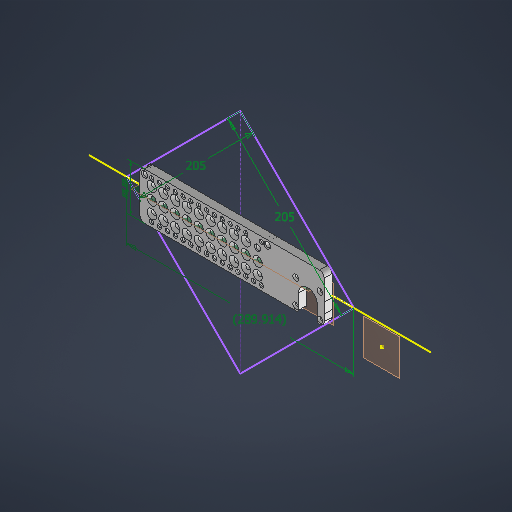
# Autodesk Inventor part: body2
Saved by Autodesk Inventor 2026.3 (Build 303398000, 398)
## iProperties
Created: 2026-04-19
Part Number: body2
Material: Generic
Document SubType Name: Modeling
Designer: micha
Density: 1 g/cm^3
Appearance: Default
Author: micha
Autodesk Inventor part; units mm, degrees
ref_plane "YZ Plane" through (0, 0, 0) normal (1, 0, 0) x (0, 1, 0)
ref_plane "XZ Plane" through (0, 0, 0) normal (0, 1, 0) x (-1, 0, 0)
ref_plane "XY Plane" through (0, 0, 0) normal (0, 0, 1) x (1, 0, 0)
ref_plane "Work Plane1" through (0, 0, 0) normal (0, 0, 1) x (1, 0, 0)
ref_plane "Work Plane2" through (-84.3749, 16.638, 0) normal (0, 0, 1) x (1, 0, 0)
sketch "Sketch2" plane through (-84.3749, 16.638, 0) normal (0, 0, 1) x (1, 0, 0)
  circle A0 centre (0, 0) radius 12
  arc A1 (21, 16.7929) -> (20.8536, 17.1464) centre (20.5, 16.7929) ccw projected
  line L0 (17.1464, 20.8536) -> (20.8536, 17.1464) projected
  arc A2 (17.1464, 20.8536) -> (16.7929, 21) centre (16.7929, 20.5) ccw projected
  line L1 (-16.7929, 21) -> (16.7929, 21) projected
  arc A3 (-16.7929, 21) -> (-17.1464, 20.8536) centre (-16.7929, 20.5) ccw projected
  line L2 (-20.8536, 17.1464) -> (-17.1464, 20.8536) projected
  arc A4 (-20.8536, 17.1464) -> (-21, 16.7929) centre (-20.5, 16.7929) ccw projected
  line L3 (-21, -16.7929) -> (-21, 16.7929) projected
  arc A5 (-21, -16.7929) -> (-20.8536, -17.1464) centre (-20.5, -16.7929) ccw projected
  line L4 (-17.1464, -20.8536) -> (-20.8536, -17.1464) projected
  arc A6 (-17.1464, -20.8536) -> (-16.7929, -21) centre (-16.7929, -20.5) ccw projected
  line L5 (16.7929, -21) -> (-16.7929, -21) projected
  arc A7 (16.7929, -21) -> (17.1464, -20.8536) centre (16.7929, -20.5) ccw projected
  line L6 (20.8536, -17.1464) -> (17.1464, -20.8536) projected
  arc A8 (20.8536, -17.1464) -> (21, -16.7929) centre (20.5, -16.7929) ccw projected
  line L7 (21, 16.7929) -> (21, -16.7929) projected
  circle A9 centre (-15.5, -15.5) radius 1.7 projected
  circle A10 centre (0, 0) radius 12 projected
  circle A11 centre (15.5, 15.5) radius 1.7 projected
  circle A12 centre (-15.5, 15.5) radius 1.7 projected
  circle A13 centre (15.5, -15.5) radius 1.7 projected
  line L8 (14.9619, 39.0381) -> (-208.0381, 39.0381)
  line L9 (-214.0381, 33.0381) -> (-214.0381, -14.9619)
  line L10 (-208.0381, -20.9619) -> (14.9619, -20.9619)
  line L11 (20.9619, -14.9619) -> (20.9619, 33.0381)
  line L12 (-260.1436, 33.0381) -> (36.1123, 33.0381)
  line L13 (-214.0381, 39.0381) -> (-208.0381, 39.0381)
  line L14 (-208.0381, 39.0381) -> (-208.0381, 33.0381)
  line L15 (-208.0381, 33.0381) -> (-214.0381, 33.0381)
  line L16 (-214.0381, 33.0381) -> (-214.0381, 39.0381)
  circle A14 centre (-208.0381, 33.0381) radius 3
  circle A15 centre (-208.0381, 33.0381) radius 20
  circle A16 centre (0, 0) radius 22
  circle A17 centre (-51.7452, 33.0381) radius 20
  circle A18 centre (-51.7452, 33.0381) radius 3
  arc A19 (-208.0381, 39.0381) -> (-214.0381, 33.0381) centre (-208.0381, 33.0381) ccw
  arc A20 (20.9619, 33.0381) -> (14.9619, 39.0381) centre (14.9619, 33.0381) ccw
  arc A21 (-214.0381, -14.9619) -> (-208.0381, -20.9619) centre (-208.0381, -14.9619) ccw
  arc A22 (14.9619, -20.9619) -> (20.9619, -14.9619) centre (14.9619, -14.9619) ccw
  line L17 (-96.5381, -135.9188) -> (48.4188, 9.0381)
  line L18 (48.4188, 9.0381) -> (-96.5381, 153.995)
  line L19 (-96.5381, 153.995) -> (-241.495, 9.0381)
  line L20 (-241.495, 9.0381) -> (-96.5381, -135.9188)
  line L21 (-96.5381, -135.9188) -> (-96.5381, 153.995) construction
  line L22 (48.4188, 9.0381) -> (-241.495, 9.0381) construction
  line L23 (-214.0381, 9.0381) -> (178.4533, 9.0381)
  point P0 (84.3749, -16.638)
  point P1 (-214.0381, -20.9619)
  point P2 (20.9619, -20.9619)
  point P3 (-16.9842, -20.9619)
  point P4 (20.9619, 16.9842)
  point P5 (-6.6781, -20.9619)
  point P6 (6.6781, -20.9619)
  point P7 (20.9619, -6.6781)
  point P8 (21, -6.5574)
  point P9 (21, 6.5574)
  point P10 (20.9619, 6.6781)
  point P11 (-6.5574, -21)
  point P12 (6.5574, -21)
  point P13 (-96.5381, 9.0381)
  dimension "d0" = 24
  dimension "d1" = 235
  dimension "d2" = 60
  dimension "d3" = 6
  dimension "d4" = 6
  dimension "d5" = 6
  dimension "d6" = 6
  dimension "d7" = 40
  dimension "d8" = 44
  dimension "d9" = 40
  dimension "d10" = 6
  dimension "d11" = 6
  dimension "d63" = 205
  dimension "d64" = 205
  constraints: 32 end point, 10 centre point, 10 point on circle, 10 point on line, 8 tangent, 6 parallel, 4 coincident, 4 horizontal, 3 equal radius, 3 midpoint, 3 perpendicular
  measures "d0" diameter of A0
  measures "d1" distance of point (20.962, -20.962) point (-214.038, -20.962)
  measures "d2" distance of point (-214.038, -20.962) L13.start
  measures "d3" distance between parallel lines of L12 L8
  measures "d4" distance of L14.end L15.end
  measures "d5" distance of L13.end L14.end
  measures "d6" diameter of A14
  measures "d7" diameter of A15
  measures "d8" diameter of A16
  measures "d9" diameter of A17
  measures "d10" diameter of A18
  measures "d11" radius of A19
  measures "d63" distance of L19.end L18.end
  measures "d64" distance of L18.end L17.end
extrude "Extrusion1" add sketch "Sketch2" along normal blind 10 contours A0 L23 A16 L11 A13 L10 A9 L3 | A0 L23 A16 A12 L1 A11 | L23 L11 A16 | A16 A11 L1 A2 L0 A1 L11 L23 | L23 L3 A4 L2 A3 L1 A16 A12 | A16 L3 L23 | A16 L7 L11 | A16 L3 A5 L4 A6 L10 A21 L9 L23 | L3 A16 | L23 L9 A15 L12 A17 L11 A1 L0 A2 L1 A16 A3 L2 A4 L3 | L11 A22 L6 L10 A16 A13 | A16 A9 L10 A6 L4 A5 L3 | L1 A16 | L12 A17 L8 A20 | L9 L12 A14 A15 | A22 L6 | A17 L12 A18 | L12 A18 A17 L8 | A19 L14 A14 L12 | A15 L8 A17 L12 | L12 A14 L14 L8 A15 | A16 L5 L10
sketch "Sketch3" plane through (-84.3749, 16.638, 10) normal (0, 0, 1) x (1, 0, 0)
  line L0 (-214.0381, 33.0381) -> (-214.0381, -14.9619) projected
  arc A0 (-214.0381, -14.9619) -> (-208.0381, -20.9619) centre (-208.0381, -14.9619) ccw projected
  line L1 (-208.0381, -20.9619) -> (-6.6781, -20.9619) projected
  arc A1 (-6.6781, -20.9619) -> (-6.5574, -21) centre (0, 0) ccw projected
  line L2 (6.6781, -20.9619) -> (14.9619, -20.9619) projected
  arc A2 (14.9619, -20.9619) -> (20.9619, -14.9619) centre (14.9619, -14.9619) ccw projected
  line L3 (20.9619, -14.9619) -> (20.9619, -6.6781) projected
  arc A3 (20.9619, -6.6781) -> (21, -6.5574) centre (0, 0) ccw projected
  line L4 (21, -6.5574) -> (21, 6.5574) projected
  arc A4 (21, 6.5574) -> (20.9619, 6.6781) centre (0, 0) ccw projected
  line L5 (20.9619, 6.6781) -> (20.9619, 33.0381) projected
  arc A5 (20.9619, 33.0381) -> (14.9619, 39.0381) centre (14.9619, 33.0381) ccw projected
  line L6 (14.9619, 39.0381) -> (-208.0381, 39.0381) projected
  arc A6 (-208.0381, 39.0381) -> (-214.0381, 33.0381) centre (-208.0381, 33.0381) ccw projected
  circle A7 centre (-208.0381, 33.0381) radius 3 projected
  circle A8 centre (-51.7452, 33.0381) radius 3 projected
  circle A9 centre (15.5, -15.5) radius 1.7 projected
  circle A10 centre (15.5, 15.5) radius 1.7 projected
  circle A11 centre (-15.5, 15.5) radius 1.7 projected
  circle A12 centre (0, 0) radius 12 projected
  circle A13 centre (-15.5, -15.5) radius 1.7 projected
  line L7 (-254.0739, 24.0381) -> (55.8114, 24.0381)
  line L8 (47.6766, 9.0381) -> (-287.6299, 9.0381)
  line L9 (-199.0381, -79.9985) -> (-199.0381, 84.2229)
  circle A14 centre (-199.0381, 24.0381) radius 3
  line L10 (-6.5574, -21) -> (6.5574, -21) projected
  arc A15 (6.5574, -21) -> (6.6781, -20.9619) centre (0, 0) ccw projected
  point P0 (84.3749, -16.638)
  dimension "d17" = 15
  dimension "d18" = 15
  dimension "d19" = 15
  dimension "d20" = 6
  constraints: 6 end point, 2 horizontal, 2 point on line, 1 centre point, 1 vertical
  measures "d17" distance between parallel lines of L6 L7
  measures "d18" distance between parallel lines of L7 L8
  measures "d19" distance between parallel lines of L9 L0
  measures "d20" diameter of A14
extrude "Extrusion2" cut sketch "Sketch3" against normal through all contours A14 L9 L7 | L7 L9 A14 | L9 A14 L7 | L7 A14 L9
pattern_linear "Rectangular Pattern1" count 10 spacing 15 along (1, 0, 0) count 3 spacing 15 along (0, -1, 0) of "Extrusion2"
sketch "Sketch4" plane through (-84.3749, 16.638, 0) normal (0, 0, -1) x (-1, 0, 0)
  circle A0 centre (208.0381, 33.0381) radius 3 projected
  circle A1 centre (51.7452, 33.0381) radius 3 projected
  line L0 (205.1513, 28.0381) -> (202.2646, 33.0381)
  line L1 (202.2646, 33.0381) -> (205.1513, 38.0381)
  line L2 (205.1513, 38.0381) -> (210.9248, 38.0381)
  line L3 (210.9248, 38.0381) -> (213.8116, 33.0381)
  line L4 (213.8116, 33.0381) -> (210.9248, 28.0381)
  line L5 (210.9248, 28.0381) -> (205.1513, 28.0381)
  line L6 (54.6319, 38.0381) -> (57.5187, 33.0381)
  line L7 (57.5187, 33.0381) -> (54.6319, 28.0381)
  line L8 (54.6319, 28.0381) -> (48.8584, 28.0381)
  line L9 (48.8584, 28.0381) -> (45.9717, 33.0381)
  line L10 (45.9717, 33.0381) -> (48.8584, 38.0381)
  line L11 (48.8584, 38.0381) -> (54.6319, 38.0381)
  point P0 (-84.3749, -16.638)
  dimension "d29" = 10
  dimension "d30" = 10
  constraints: 24 end point, 2 coincident, 26 other
  measures "d29" distance between parallel lines of L2 L5
  measures "d30" distance between parallel lines of L11 L8
extrude "Extrusion3" cut sketch "Sketch4" against normal blind 4 contours A0 | A1 | L0 L1 L2 L3 L4 L5 | L6 L7 L8 L9 L10 L11
ref_plane "Work Plane3" through (-292.413, 25.676, 0) normal (0, -1, 0) x (1, 0, 0)
sketch "Sketch5" plane through (-84.3749, 16.638, 10) normal (0, 0, 1) x (1, 0, 0)
  circle A0 centre (-199.0381, -5.9619) radius 3 projected
  line L0 (-199.0381, -8.9619) -> (-199.0381, -20.9619)
  line L1 (-208.0381, -20.9619) -> (-6.6781, -20.9619) projected
  line L2 (-199.0381, -14.9619) -> (37.7784, -14.9619)
  circle A1 centre (-199.0381, -14.9619) radius 1.85
  circle A2 centre (-189.0381, -14.9619) radius 1.85
  circle A3 centre (-179.0381, -14.9619) radius 1.85
  circle A4 centre (-169.0381, -14.9619) radius 1.85
  circle A5 centre (-159.0381, -14.9619) radius 1.85
  circle A6 centre (-149.0381, -14.9619) radius 1.85
  circle A7 centre (-139.0381, -14.9619) radius 1.85
  circle A8 centre (-129.0381, -14.9619) radius 1.85
  circle A9 centre (-119.0381, -14.9619) radius 1.85
  circle A10 centre (-109.0381, -14.9619) radius 1.85
  circle A11 centre (-99.0381, -14.9619) radius 1.85
  circle A12 centre (-89.0381, -14.9619) radius 1.85
  circle A13 centre (-79.0381, -14.9619) radius 1.85
  circle A14 centre (-69.0381, -14.9619) radius 1.85
  circle A15 centre (-59.0381, -14.9619) radius 1.85
  line L3 (-214.0381, 33.0381) -> (-214.0381, -14.9619) projected
  line L4 (-214.0381, 9.0381) -> (17.5819, 9.0381)
  line L5 (-199.0381, 27.0381) -> (-199.0381, 39.0381)
  line L6 (-199.0381, 33.0381) -> (37.7784, 33.0381)
  circle A16 centre (-199.0381, 33.0381) radius 1.85
  circle A17 centre (-189.0381, 33.0381) radius 1.85
  circle A18 centre (-179.0381, 33.0381) radius 1.85
  circle A19 centre (-169.0381, 33.0381) radius 1.85
  circle A20 centre (-159.0381, 33.0381) radius 1.85
  circle A21 centre (-149.0381, 33.0381) radius 1.85
  circle A22 centre (-139.0381, 33.0381) radius 1.85
  circle A23 centre (-129.0381, 33.0381) radius 1.85
  circle A24 centre (-119.0381, 33.0381) radius 1.85
  circle A25 centre (-109.0381, 33.0381) radius 1.85
  circle A26 centre (-99.0381, 33.0381) radius 1.85
  circle A27 centre (-89.0381, 33.0381) radius 1.85
  circle A28 centre (-79.0381, 33.0381) radius 1.85
  circle A29 centre (-69.0381, 33.0381) radius 1.85
  circle A30 centre (-59.0381, 33.0381) radius 1.85
  point P0 (84.3749, -16.638)
  dimension "d33" = 3.7
  dimension "d36" = 10
  constraints: 30 centre point, 19 symmetric about line, 10 end point, 3 horizontal, 2 coincident, 2 midpoint, 1 point on line, 1 vertical, 1 vertical alignment, 44 other
  measures "d33" diameter of A1
  measures "d36" distance of A1.centre A2.centre
extrude "Extrusion4" cut sketch "Sketch5" against normal through all contours A1 L2 L0 | L0 A1 | L2 A1 L0 | A2 L2 | L2 A2 | A3 L2 | L2 A3 | A4 L2 | L2 A4 | A5 L2 | L2 A5 | A6 L2 | L2 A6 | A7 L2 | L2 A7 | A8 L2 | L2 A8 | A9 L2 | L2 A9 | A10 L2 | L2 A10 | A11 L2 | L2 A11 | A12 L2 | L2 A12 | A13 L2 | L2 A13 | A14 L2 | L2 A14 | A15 L2 | L2 A15 | A16 L5 | L5 L6 A16 | L5 A16 L6 | A17 L6 | L6 A17 | A18 L6 | L6 A18 | A19 L6 | L6 A19 | A20 L6 | L6 A20 | A21 L6 | L6 A21 | A22 L6 | L6 A22 | A23 L6 | L6 A23 | A24 L6 | L6 A24 | A25 L6 | L6 A25 | A26 L6 | L6 A26 | A27 L6 | L6 A27 | A28 L6 | L6 A28 | A30 L6 | L6 A30
sketch "Sketch6" plane through (-84.3749, 16.638, 10) normal (0, 0, 1) x (1, 0, 0)
  circle A0 centre (0, 0) radius 12 projected
  line L0 (12, 0) -> (-12, 0)
  line L1 (-12, 0) -> (-12, -28.4765)
  line L2 (-12, -28.4765) -> (12, -28.4765)
  line L3 (12, -28.4765) -> (12, 0)
  point P0 (84.3749, -16.638)
  point P1 (-12, 0)
  constraints: 8 end point, 2 parallel, 1 horizontal, 1 perpendicular, 2 other
extrude "Extrusion5" cut sketch "Sketch6" against normal through all contours L3 L2 L1 A0
fillet "Fillet1" radius 2 2 edges at (-96.3749, -4.324, 5) (-72.3749, -4.324, 5)
chamfer "Chamfer1" distance 2 angle 45 4 edges at (-101.5749, 1.138, 10) (-101.5749, 32.138, 10) (-70.5749, 32.138, 10) (-70.5749, 1.138, 10)
chamfer "Chamfer3" distance 1 angle 45 32 edges at (-285.263, 1.676, 10) (-275.263, 1.676, 10) (-265.263, 1.676, 10) (-255.263, 1.676, 10) (-245.263, 1.676, 10) (-235.263, 1.676, 10) (-225.263, 1.676, 10) (-215.263, 1.676, 10) (-205.263, 1.676, 10) (-195.263, 1.676, 10) (-185.263, 1.676, 10) (-175.263, 1.676, 10) (-165.263, 1.676, 10) (-155.263, 1.676, 10) (-145.263, 1.676, 10) (-165.263, 49.676, 10) (-145.263, 49.676, 10) (-175.263, 49.676, 10) (-185.263, 49.676, 10) (-195.263, 49.676, 10) (-205.263, 49.676, 10) (-215.263, 49.676, 10) (-225.263, 49.676, 10) (-235.263, 49.676, 10) (-245.263, 49.676, 10) (-255.263, 49.676, 10) (-265.263, 49.676, 10) (-275.263, 49.676, 10) (-285.263, 49.676, 10) (-295.413, 49.676, 10) (-139.1201, 49.676, 10) (-151.413, 40.676, 10)
chamfer "Chamfer4" distance 1 angle 45 28 edges at (-285.263, 1.676, 0) (-275.263, 1.676, 0) (-265.263, 1.676, 0) (-255.263, 1.676, 0) (-245.263, 1.676, 0) (-235.263, 1.676, 0) (-225.263, 1.676, 0) (-215.263, 1.676, 0) (-205.263, 1.676, 0) (-195.263, 1.676, 0) (-285.263, 49.676, 0) (-275.263, 49.676, 0) (-265.263, 49.676, 0) (-255.263, 49.676, 0) (-245.263, 49.676, 0) (-165.263, 49.676, 0) (-175.263, 49.676, 0) (-185.263, 49.676, 0) (-195.263, 49.676, 0) (-205.263, 49.676, 0) (-215.263, 49.676, 0) (-225.263, 49.676, 0) (-235.263, 49.676, 0) (-145.263, 1.676, 0) (-155.263, 1.676, 0) (-165.263, 1.676, 0) (-175.263, 1.676, 0) (-185.263, 1.676, 0)
chamfer "Chamfer5" distance 3 angle 45 29 edges at (-286.413, 10.676, 10) (-286.413, 25.676, 10) (-286.413, 40.676, 10) (-271.413, 40.676, 10) (-271.413, 25.676, 10) (-271.413, 10.676, 10) (-256.413, 10.676, 10) (-256.413, 25.676, 10) (-256.413, 40.676, 10) (-241.413, 25.676, 10) (-241.413, 10.676, 10) (-241.413, 40.676, 10) (-226.413, 40.676, 10) (-226.413, 25.676, 10) (-226.413, 10.676, 10) (-211.413, 10.676, 10) (-211.413, 25.676, 10) (-211.413, 40.676, 10) (-196.413, 40.676, 10) (-196.413, 25.676, 10) (-196.413, 10.676, 10) (-181.413, 10.676, 10) (-166.413, 10.676, 10) (-151.413, 10.676, 10) (-151.413, 25.676, 10) (-166.413, 25.676, 10) (-181.413, 25.676, 10) (-181.413, 40.676, 10) (-166.413, 40.676, 10)
sketch "Sketch7" plane through (-84.3749, 16.638, 0) normal (0, 0, -1) x (-1, 0, 0)
  line L0 (96.0895, -135.9188) -> (241.0464, 9.0381)
  line L1 (241.0464, 9.0381) -> (96.0895, 153.995)
  line L2 (96.0895, 153.995) -> (-48.8673, 9.0381)
  line L3 (-48.8673, 9.0381) -> (96.0895, -135.9188)
  line L4 (96.0895, -135.9188) -> (96.0895, 153.995) construction
  line L5 (241.0464, 9.0381) -> (-48.8673, 9.0381) construction
  line L6 (241.0464, 9.0381) -> (-48.8673, 9.0381)
  line L7 (288.617, 9.0381) -> (-146.5403, 9.0381) projected
  line L8 (214.0381, 33.0381) -> (214.0381, -14.9619) projected
  point P0 (-84.3749, -16.638)
  point P1 (96.0895, 9.0381)
  point P2 (214.0381, 9.0381)
  dimension "d61" = 205
  dimension "d62" = 205
  dimension "d65" = 289.9138
  constraints: 14 end point, 3 equal length, 3 midpoint, 2 point on line, 1 perpendicular
  measures "d61" distance of L2.end L1.end
  measures "d62" distance of L1.end L0.end
  measures "d65" distance of L2.end L0.end
body "Solid1"
